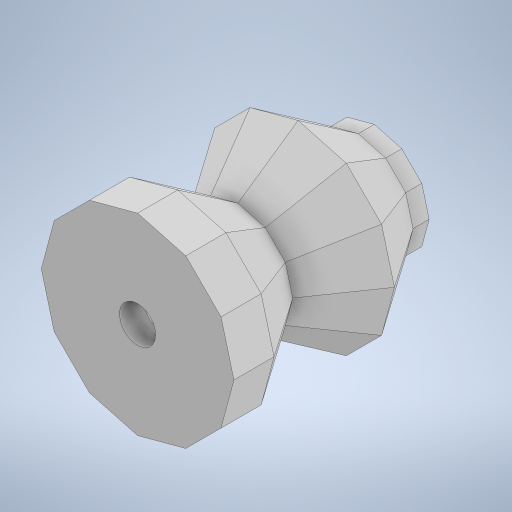
# Autodesk Inventor part: Test15
Saved by Autodesk Inventor 2023 (Build 270158000, 158)
## iProperties
Created: 2024-07-02
Part Number: Test15
Material: 일반
Document SubType Name: Modeling
Designer: ojs08
Density: 1 g/cm^3
Appearance: 기본값
Author: ojs08
Autodesk Inventor part; units mm, degrees
ref_plane "YZ Plane" through (0, 0, 0) normal (1, 0, 0) x (0, 1, 0)
ref_plane "XZ Plane" through (0, 0, 0) normal (0, 1, 0) x (-1, 0, 0)
ref_plane "XY Plane" through (0, 0, 0) normal (0, 0, 1) x (1, 0, 0)
sketch "스케치1" plane through (0, 0, 0) normal (0, 0, 1) x (1, 0, 0)
  circle A0 centre (0, 0) radius 12
  line L0 (12, 0) -> (10.3923, -6)
  line L1 (10.3923, -6) -> (6, -10.3923)
  line L2 (6, -10.3923) -> (0, -12)
  line L3 (0, -12) -> (-6, -10.3923)
  line L4 (-6, -10.3923) -> (-10.3923, -6)
  line L5 (-10.3923, -6) -> (-12, 0)
  line L6 (-12, 0) -> (-10.3923, 6)
  line L7 (-10.3923, 6) -> (-6, 10.3923)
  line L8 (-6, 10.3923) -> (0, 12)
  line L9 (0, 12) -> (6, 10.3923)
  line L10 (6, 10.3923) -> (10.3923, 6)
  line L11 (10.3923, 6) -> (12, 0)
  dimension "d0" = 24
  constraints: 24 end point, 2 coincident, 1 horizontal alignment, 27 other
extrude "돌출1" add sketch "스케치1" along normal blind 7.5 draft -33.69 contours L0 L1 L2 L3 L4 L5 L6 L7 L8 L9 L10 L11
mirror "미러1" about plane through (0, 0, 7.5) normal (0, 0, 1) of "돌출1"
mirror "미러2" about plane through (0, 0, 0) normal (0, 0, -1) of "돌출1"
sketch "스케치2" plane through (6.8236, 0, -7.5) normal (0, 0, -1) x (-0.9659258, -0.258819, 0)
  point P0 (6.5911, 1.7661)
sketch "스케치3" plane through (10.3923, 6, 15) normal (0, 0, 1) x (0.7071068, 0.7071068, 0)
  point P0 (-11.5911, 3.1058)
sketch "스케치8" plane through (10.3923, 6, 15) normal (0, 0, 1) x (0.7071068, 0.7071068, 0)
  line L0 (0, 0) -> (0, 6.2117) projected
  line L1 (0, 6.2117) -> (-3.1058, 11.5911) projected
  line L2 (-3.1058, 11.5911) -> (-8.4853, 14.6969) projected
  line L3 (-8.4853, 14.6969) -> (-14.6969, 14.6969) projected
  line L4 (-14.6969, 14.6969) -> (-20.0764, 11.5911) projected
  line L5 (-20.0764, 11.5911) -> (-23.1822, 6.2117) projected
  line L6 (-23.1822, 6.2117) -> (-23.1822, 0) projected
  line L7 (-23.1822, 0) -> (-20.0764, -5.3795) projected
  line L8 (-20.0764, -5.3795) -> (-14.6969, -8.4853) projected
  line L9 (-14.6969, -8.4853) -> (-8.4853, -8.4853) projected
  line L10 (-8.4853, -8.4853) -> (-3.1058, -5.3795) projected
  line L11 (-3.1058, -5.3795) -> (0, 0) projected
  point P0 (-11.5911, 3.1058)
extrude "돌출6" add sketch "스케치8" along normal blind 2.5
shell "쉘2" thickness 0.5 removed faces 0 ; own thickness 2 on faces at (-9.7386, 2, -2.5) (-6.6014, 7.4339, -2.5) (-3.1373, 9.4339, -2.5) (2, 9.7386, -2.5) (7.4339, 6.6014, -2.5) (-2, -9.7386, -2.5) (2, -9.7386, -2.5) (6.6014, -7.4339, -2.5) (9.4339, -3.1373, -2.5) (9.7386, 2, -2.5) (-6.6014, -7.4339, -2.5) (-9.7386, -2, -2.5) (7.4339, 6.6014, 12.5) (2, 9.7386, 12.5) (-2, 9.7386, 12.5) (9.7386, 2, 12.5) (9.4339, -3.1373, 12.5) (6.6014, -7.4339, 12.5) (2, -9.7386, 12.5) (-3.1373, -9.4339, 12.5) (-7.4339, -6.6014, 12.5) (-6.6014, 7.4339, 12.5) (-9.4339, 3.1373, 12.5) (-9.7386, -2, 12.5)
sketch "스케치9" plane through (10.3923, 6, 17.5) normal (0, 0, 1) x (0.7071068, -0.7071068, 0)
  line L0 (-6.2117, 0) -> (-11.5911, -3.1058) projected
  line L1 (-11.5911, -3.1058) -> (-14.6969, -8.4853) projected
  line L2 (-14.6969, -8.4853) -> (-14.6969, -14.6969) projected
  line L3 (-14.6969, -14.6969) -> (-11.5911, -20.0764) projected
  line L4 (-11.5911, -20.0764) -> (-6.2117, -23.1822) projected
  line L5 (-6.2117, -23.1822) -> (0, -23.1822) projected
  line L6 (0, -23.1822) -> (5.3795, -20.0764) projected
  line L7 (5.3795, -20.0764) -> (8.4853, -14.6969) projected
  line L8 (8.4853, -14.6969) -> (8.4853, -8.4853) projected
  line L9 (8.4853, -8.4853) -> (5.3795, -3.1058) projected
  line L10 (5.3795, -3.1058) -> (0, 0) projected
  line L11 (0, 0) -> (-6.2117, 0) projected
  point P0 (-3.1058, -11.5911)
extrude "돌출7" add sketch "스케치9" along normal blind 2.5
sketch "스케치10" plane through (10.3923, 6, 20) normal (0, 0, 1) x (0.7071068, 0.7071068, 0)
  circle A0 centre (-11.5911, 3.1058) radius 2.25
  dimension "d20" = 4.5
  constraints: 1 centre point, 1 coincident
  measures "d20" diameter of A0
extrude "돌출8" cut sketch "스케치10" against normal blind 3
sketch "스케치11" plane through (6.8236, 0, -7.5) normal (0, 0, -1) x (-0.9659258, -0.258819, 0)
  line L0 (0, 3.5322) -> (0, 0) projected
  line L1 (0, 0) -> (1.7661, -3.059) projected
  line L2 (1.7661, -3.059) -> (4.825, -4.825) projected
  line L3 (4.825, -4.825) -> (8.3572, -4.825) projected
  line L4 (8.3572, -4.825) -> (11.4162, -3.059) projected
  line L5 (11.4162, -3.059) -> (13.1822, 0) projected
  line L6 (13.1822, 0) -> (13.1822, 3.5322) projected
  line L7 (13.1822, 3.5322) -> (11.4162, 6.5911) projected
  line L8 (11.4162, 6.5911) -> (8.3572, 8.3572) projected
  line L9 (8.3572, 8.3572) -> (4.825, 8.3572) projected
  line L10 (4.825, 8.3572) -> (1.7661, 6.5911) projected
  line L11 (1.7661, 6.5911) -> (0, 3.5322) projected
  point P0 (6.5911, 1.7661)
extrude "돌출9" add sketch "스케치11" along normal blind 2
